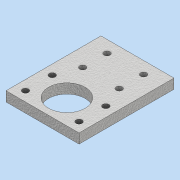
# Autodesk Inventor part: Uchwyt silnika krokowego osi Y - płaski
Saved by Autodesk Inventor 2018 (Build 220112000, 112)
## iProperties
Created: 2019-01-31
Part Number: Uchwyt silnika krokowego osi Y - płaski
Material: Ogólny
Document SubType Name: Modeling
Designer: Dawid
Density: 1 g/cm^3
Appearance: Aluminium odlewane
Author: Dawid
Autodesk Inventor part; units mm, degrees
ref_plane "YZ Plane" through (0, 0, 0) normal (1, 0, 0) x (0, 1, 0)
ref_plane "XZ Plane" through (0, 0, 0) normal (0, 1, 0) x (-1, 0, 0)
ref_plane "XY Plane" through (0, 0, 0) normal (0, 0, 1) x (1, 0, 0)
sketch "Szkic1" plane through (0, 0, 0) normal (0, 0, 1) x (1, 0, 0)
  line L0 (-30, 58) -> (30, 58)
  circle A0 centre (0, 0) radius 15
  line L1 (0, 0) -> (30, 0)
  line L2 (30, 0) -> (30, 58)
  line L3 (-30, 0) -> (-30, 58)
  line L4 (-30, 0) -> (-30, -20)
  line L5 (-30, -20) -> (30, -20)
  line L6 (30, -20) -> (30, 0)
  dimension "d2" = 30
  dimension "d7" = 78
  dimension "d8" = 60
  dimension "d9" = 20
  constraints: 14 end point, 4 perpendicular, 3 point on line, 1 centre point, 1 horizontal
  measures "d2" diameter of A0
  measures "d7" distance between parallel lines of L5 L0
  measures "d8" distance of L0.start L0.end
  measures "d9" distance from line of L5 point (0, 0)
extrude "Wyciągnięcie proste1" add sketch "Szkic1" along normal blind 8
sketch "Szkic2" plane through (0, 0, 8) normal (0, 0, 1) x (1, 0, 0)
  line L0 (30, 58) -> (-30, 58) projected
  line L1 (-30, 58) -> (-30, 18)
  line L2 (-30, 58) -> (-30, -20) projected
  line L3 (-30, 18) -> (30, 18)
  line L4 (30, -20) -> (30, 58) projected
  line L5 (30, 18) -> (30, 58)
  line L6 (-30, 58) -> (-30, 48)
  line L7 (-30, 18) -> (-30, 28)
  line L8 (-30, 28) -> (30, 28)
  line L9 (-30, 48) -> (30, 48)
  line L10 (-30, 48) -> (-15, 48)
  line L11 (-15, 48) -> (-15, 28)
  line L12 (30, 48) -> (15, 48)
  line L13 (15, 48) -> (15, 28)
  circle A0 centre (-15, 48) radius 2.5
  circle A1 centre (15, 48) radius 2.5
  circle A2 centre (-15, 28) radius 2.5
  circle A3 centre (15, 28) radius 2.5
  point P0 (0, 0)
  dimension "d12" = 40
  dimension "d13" = 90
  dimension "d14" = 10
  dimension "d15" = 10
  dimension "d16" = 15
  dimension "d17" = 15
  dimension "d18" = 5
  dimension "d19" = 5
  dimension "d20" = 5
  dimension "d21" = 5
  constraints: 22 end point, 10 point on line, 4 centre point, 4 coincident, 3 perpendicular, 1 parallel
  measures "d12" distance of L0.end L1.end
  measures "d13" angle of L3 L1
  measures "d14" distance of L0.end L6.end
  measures "d15" distance of L1.end L7.end
  measures "d16" distance of L6.end L10.end
  measures "d17" distance of L9.end L12.end
  measures "d18" diameter of A0
  measures "d19" diameter of A1
  measures "d20" diameter of A2
  measures "d21" diameter of A3
extrude "Wyciągnięcie proste2" cut sketch "Szkic2" against normal up to next contours A1 L13 L9 | L9 A1 | A0 L9 | L9 L11 A0 | A3 L8 | L8 L13 A3 | L13 A1 L9 | A2 L11 L8 | L8 A2 | L9 A0 L11 | L8 A3 L13 | L11 A2 L8
sketch "Szkic3" plane through (0, 0, 0) normal (0, 0, -1) x (-1, 0, 0)
  circle A0 centre (0, 0) radius 15
  line L0 (-30, -20) -> (30, -20)
  line L1 (30, -20) -> (30, 18)
  line L2 (30, 18) -> (-30, 18)
  line L3 (-30, 18) -> (-30, -20)
  line L4 (-30, 18) -> (-30, -20)
  line L5 (-30, 18) -> (-22, 18)
  line L6 (30, 18) -> (-30, 18)
  line L7 (-22, 18) -> (-22, -20)
  line L8 (30, 18) -> (22, 18)
  line L9 (22, 18) -> (22, -20)
  line L10 (-22, 18) -> (-22, 10)
  line L11 (-22, -20) -> (-22, -12)
  line L12 (22, 18) -> (22, 10)
  line L13 (22, -20) -> (22, -12)
  circle A1 centre (-22, 10) radius 2.5
  circle A2 centre (-22, -12) radius 2.5
  circle A3 centre (22, 10) radius 2.5
  circle A4 centre (22, -12) radius 2.5
  circle A5 centre (-15, 28) radius 2.5 projected
  circle A6 centre (-15, 48) radius 2.5 projected
  circle A7 centre (15, 48) radius 2.5 projected
  circle A8 centre (15, 28) radius 2.5 projected
  circle A9 centre (0, 0) radius 15 projected
  line L14 (30, 58) -> (-30, 58) projected
  line L15 (-30, 58) -> (-30, -20) projected
  line L16 (-30, -20) -> (30, -20) projected
  line L17 (30, -20) -> (30, 58) projected
  point P0 (0, -1)
  dimension "d24" = 8
  dimension "d25" = 8
  dimension "d26" = 8
  dimension "d27" = 8
  dimension "d28" = 8
  dimension "d29" = 8
  dimension "d30" = 5
  dimension "d31" = 5
  dimension "d32" = 5
  dimension "d33" = 5
  constraints: 28 end point, 8 point on line, 5 centre point, 4 coincident, 2 perpendicular
  measures "d24" distance of L2.end L5.end
  measures "d25" distance of L1.end L8.end
  measures "d26" distance of L5.end L10.end
  measures "d27" distance of L7.end L11.end
  measures "d28" distance of L8.end L12.end
  measures "d29" distance of L9.end L13.end
  measures "d30" diameter of A1
  measures "d31" diameter of A2
  measures "d32" diameter of A3
  measures "d33" diameter of A4
extrude "Wyciągnięcie proste3" cut sketch "Szkic3" against normal up to next contours A2 L7 | L7 A2 | A4 L9 | L9 A4 | A1 L7 | L7 A1 | A3 L9 | L9 A3
thread "Gwint1" size "M5x0.8" class "6H" standard "ANSI Metric M Profile" full length
thread "Gwint2" size "M5x0.8" class "6H" standard "ANSI Metric M Profile" full length
thread "Gwint3" size "M5x0.8" class "6H" standard "ANSI Metric M Profile" full length
thread "Gwint4" size "M5x0.8" class "6H" standard "ANSI Metric M Profile" full length
